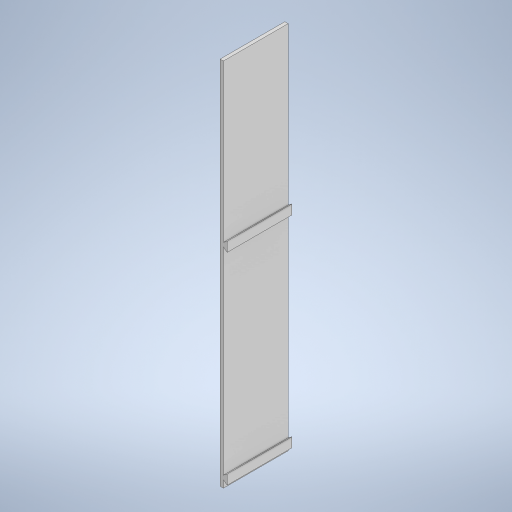
# Autodesk Inventor part: guide_ver2
Saved by Autodesk Inventor 2024 (Build 280153000, 153)
## iProperties
Created: 2023-11-13
Part Number: guide_ver2
Material: 一般
Document SubType Name: Modeling
Designer: Kota Taga
Density: 1 g/cm^3
Appearance: 既定
Author: Kota Taga
## iProperties of the stored document guide_3D プリント.ipt
Created: 2023-11-13
Part Number: guide_3D プリント
Material: 一般
Document SubType Name: Modeling
Designer: Kota Taga
Density: 1 g/cm^3
Appearance: 既定
Author: Kota Taga
Autodesk Inventor part; units mm, degrees
ref_plane "YZ Plane" through (0, 0, 0) normal (1, 0, 0) x (0, 1, 0)
ref_plane "XZ Plane" through (0, 0, 0) normal (0, 1, 0) x (-1, 0, 0)
ref_plane "XY Plane" through (0, 0, 0) normal (0, 0, 1) x (1, 0, 0)
sketch "スケッチ1" plane through (0, 0, 0) normal (0, 1, 0) x (-1, 0, 0)
  line L0 (1, 17.5) -> (-1, 17.5)
  line L1 (-1, 17.5) -> (-1, -17.5)
  line L2 (-1, -17.5) -> (1, -17.5)
  line L3 (1, -17.5) -> (1, 17.5)
  line L4 (1.4, 0) -> (-1.4, 0) projected
  line L5 (0, -24.5) -> (0, 24.5) projected
  point P0 (0, 0)
  dimension "d0" = 2
  dimension "d1" = 35
  constraints: 8 end point, 2 parallel, 1 horizontal, 1 perpendicular, 2 other
  measures "d0" distance of L1.end L2.end
  measures "d1" distance of L2.end L0.start
extrude "押し出し1" add sketch "スケッチ1" along normal blind 200
sketch "スケッチ4" plane through (1, 0, 17.5) normal (0, 0, 1) x (1, 0, 0)
  line L0 (0, 0) -> (0, 200) projected
  line L1 (0, 2) -> (2, 2)
  line L2 (2, 2) -> (2, 8)
  line L3 (2, 8) -> (0, 8)
  line L4 (0, 8) -> (0, 2)
  line L5 (-2, 0) -> (0, 0) projected
  line L6 (0, 6.5) -> (2, 8)
  line L7 (0, 3.5) -> (2, 2)
  line L8 (0, 111) -> (2, 111)
  line L9 (2, 111) -> (2, 117)
  line L10 (2, 117) -> (0, 117)
  line L11 (0, 117) -> (0, 111)
  line L12 (2, 117) -> (0, 115.5)
  line L13 (2, 111) -> (0, 112.5)
  line L14 (2.12, 116.84) -> (0.12, 115.34)
  line L15 (2.12, 111.16) -> (0, 112.75)
  line L16 (1.8, 111) -> (1.8, 117)
  line L17 (0.12, 115.34) -> (0, 115.25)
  line L18 (0, 112.75) -> (0, 106.75)
  line L19 (0.12, 6.34) -> (2.12, 7.84)
  line L20 (0.12, 3.66) -> (2.12, 2.16)
  line L21 (1.8, 2) -> (1.8, 8)
  line L22 (0.12, 6.34) -> (0, 6.25)
  line L23 (0.12, 3.66) -> (0, 3.75)
  point P0 (-1, 0)
  point P1 (0, 3.75)
  point P2 (1.8, 2.4)
  point P3 (1.8, 7.6)
  point P4 (0, 6.25)
  point P5 (0, 106.75)
  point P6 (1.8, 111.4)
  point P7 (1.8, 116.6)
  point P8 (0, 115.25)
  point P9 (1, 8)
  point P10 (0, 112.75)
  dimension "d13" = 2
  dimension "d14" = 6
  dimension "d15" = 2
  dimension "d16" = 1.5
  dimension "d17" = 1.5
  dimension "d19" = 6
  dimension "d20" = 2
  dimension "d21" = 1.5
  dimension "d22" = 1.5
  dimension "d23" = 0.2
  dimension "d24" = 0.2
  dimension "d25" = 0.2
  dimension "d26" = 0.2
  dimension "d27" = 0.2
  dimension "d28" = 0.2
  dimension "d31" = 103
  dimension "d32" = 180
  constraints: 44 end point, 11 parallel, 10 point on line, 2 horizontal, 2 perpendicular, 1 midpoint
  measures "d13" distance of L2.end L3.end
  measures "d14" distance of L1.end L2.end
  measures "d15" distance between parallel lines of L5 L1
  measures "d16" distance from line of L3 L6.start
  measures "d17" distance from line of L7.start L1
  measures "d19" distance of L8.end L9.end
  measures "d20" distance of L8.start L8.end
  measures "d21" distance of L12.end L10.end
  measures "d22" distance of L8.start L13.end
  measures "d23" distance between parallel lines of L12 L14
  measures "d24" distance between parallel lines of L13 L15
  measures "d25" distance between parallel lines of L9 L16
  measures "d26" distance between parallel lines of L6 L19
  measures "d27" distance between parallel lines of L7 L20
  measures "d28" distance between parallel lines of L2 L21
  measures "d31" distance from line of point (1, 8) L8
  measures "d32" angle of L11 L18
extrude "押し出し3" add sketch "スケッチ4" against normal up to surface (35 mm away) contours L0 L22 L19 L21 L20 L23 | L0 L17 L14 L16 L15
sketch "スケッチ7" plane through (-1, 0, -17.5) normal (0, 0, -1) x (-1, 0, 0)
  line L0 (-2, 115.25) -> (-2, 200) projected
  line L1 (-2, 0) -> (0, 0) projected
  line L2 (-2, 200) -> (-1.8, 200)
  line L3 (-1.8, 200) -> (-1.8, 0)
  line L4 (-1.8, 0) -> (-2, 0)
  line L5 (-2, 0) -> (-2, 200)
  line L6 (-2, 3.75) -> (-3.8, 2.4) projected
  line L7 (-2, 3.75) -> (-1.8, 3.9)
  line L8 (-3.8, 7.6) -> (-2, 6.25) projected
  line L9 (-2, 6.25) -> (-1.8, 6.1)
  line L10 (-3.8, 116.6) -> (-2, 115.25) projected
  line L11 (-2, 115.25) -> (-1.8, 115.1)
  line L12 (-3.8, 116.6) -> (-2, 115.25) projected
  line L13 (-2, 112.75) -> (-3.8, 111.4) projected
  line L14 (-2, 112.75) -> (-1.8, 112.9)
  point P0 (-1, 0)
  dimension "d38" = 0.2
  constraints: 16 end point, 5 point on line, 4 collinear, 2 parallel, 1 horizontal, 1 perpendicular
  measures "d38" distance of L3.end L4.end
extrude "押し出し5" cut sketch "スケッチ7" against normal up to surface (35 mm away) contours L0 L2 L3 L11 | L14 L3 L9 L5 | L7 L3 L1 L5
